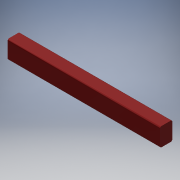
# Autodesk Inventor part: Beam
Saved by Autodesk Inventor 2019 (Build 230136000, 136)
## iProperties
Created: 2020-02-21
Part Number: Beam
Material: Generic
Document SubType Name: Modeling
Designer: ntb11189
Density: 1 g/cm^3
Appearance: Smooth - Burnt Red
Author: ntb11189
Autodesk Inventor part; units mm, degrees
ref_plane "YZ Plane" through (0, 0, 0) normal (1, 0, 0) x (0, 1, 0)
ref_plane "XZ Plane" through (0, 0, 0) normal (0, 1, 0) x (-1, 0, 0)
ref_plane "XY Plane" through (0, 0, 0) normal (0, 0, 1) x (1, 0, 0)
sketch "Sketch1" plane through (0, 0, 0) normal (1, 0, 0) x (0, 1, 0)
  line L0 (-10, 0) -> (-111, 0)
  line L1 (-121, -10) -> (-121, -71)
  line L2 (-111, -81) -> (-10, -81)
  line L3 (0, -71) -> (0, -10)
  arc A0 (0, -10) -> (-10, 0) centre (-10, -10) ccw
  arc A1 (-10, -81) -> (0, -71) centre (-10, -71) ccw
  arc A2 (-121, -71) -> (-111, -81) centre (-111, -71) ccw
  arc A3 (-111, 0) -> (-121, -10) centre (-111, -10) ccw
  point P0 (0, 0)
  point P1 (-121, -81)
  point P2 (0, -81)
  dimension "d0" = 121
  dimension "d1" = 81
  dimension "d2" = 10
  constraints: 8 end point, 8 point on circle, 8 tangent, 6 point on line, 4 centre point, 3 equal radius, 2 parallel, 1 horizontal, 1 perpendicular
  measures "d0" distance of point (0, -81) point (-121, -81)
  measures "d1" distance of point (0, -81) point (0, 0)
  measures "d2" radius of A0
extrude "Extrusion1" add sketch "Sketch1" along normal mid plane 1000
body "Solid1"
